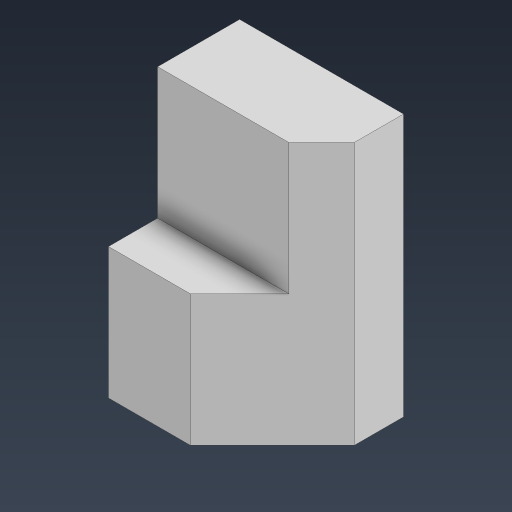
# Autodesk Inventor part: 3D Model
Saved by Autodesk Inventor 2024 (Build 280153000, 153)
## iProperties
Created: 2024-03-05
Part Number: 3D Model
Material: Genérico
Document SubType Name: Modeling
Designer: Administrator
Density: 1 g/cm^3
Appearance: Padrão
Author: Administrator
Autodesk Inventor part; units mm, degrees
ref_plane "YZ Plane" through (0, 0, 0) normal (1, 0, 0) x (0, 1, 0)
ref_plane "XZ Plane" through (0, 0, 0) normal (0, 1, 0) x (-1, 0, 0)
ref_plane "XY Plane" through (0, 0, 0) normal (0, 0, 1) x (1, 0, 0)
sketch "Esboço1" plane through (0, 0, 0) normal (0, 1, 0) x (-1, 0, 0)
  line L0 (-25, 20) -> (25, 20)
  line L1 (25, 20) -> (25, -20)
  line L2 (25, -20) -> (-25, -20)
  line L3 (-25, -20) -> (-25, 20)
  line L4 (-25, 20) -> (25, -20) construction
  line L5 (25, 20) -> (-25, -20) construction
  point P0 (0, 0)
  dimension "d0" = 50
  dimension "d1" = 40
  constraints: 12 end point, 2 midpoint, 2 parallel, 1 horizontal, 1 perpendicular
  measures "d0" distance of L1.end L2.end
  measures "d1" distance of L0.end L1.end
extrude "Extrusão1" add sketch "Esboço1" along normal blind 80
sketch "Esboço2" plane through (25, 0, 20) normal (1, 0, 0) x (0, 0, -1)
  line L0 (0, 80) -> (15, 80)
  line L1 (15, 80) -> (15, 40)
  line L2 (15, 40) -> (0, 40)
  line L3 (0, 40) -> (0, 80)
  line L4 (40, 0) -> (40, 80) projected
  line L5 (0, 0) -> (40, 0) projected
  point P0 (20, 0)
  dimension "d4" = 25
  dimension "d5" = 40
  constraints: 8 end point, 2 parallel, 1 coincident, 1 horizontal, 1 perpendicular
  measures "d4" distance between parallel lines of L4 L1
  measures "d5" distance between parallel lines of L5 L2
extrude "Extrusão2" cut sketch "Esboço2" against normal through all
chamfer "Chanfro1" distance 25 angle 45 1 edges at (25, 20, 20)
